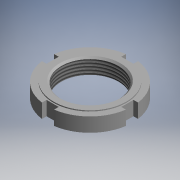
# Autodesk Inventor part: 3753 M30x1.5
Saved by Autodesk Inventor 2017.3 (Build 213256000, 256)
## iProperties
Part Number: 3753 M30x1.5
Material: Generic
Catalog Web Link: www.cadenas.de
Description: NUT-SLOTTED-Slotted nut
Vendor: FESTO
Document SubType Name: Modeling
Designer: partserver
Manufacturer: FESTO
Mass: 5.20156 g
Surface Area: 31.9496 cm^2
Volume: 5.20156 cm^3
Density: 1 g/cm^3
Appearance: PSOLRGB-192-192-192
Category: PARTsolutions
Company: FESTO
Title: 3753 M30x1.5
Author: Cadenas PARTsolutions
Comments: Slotted nut
PSOL_IDENT_0: {$CADENAS_DATA\23d-libs\festo\zyl_zubeh\nutmutter\slotted_nut.prj},169 {VTYP=3D},{NB=3753 M30x1.5},{
PSOL_IDENT_1: LINA=3753 M30x1.5},{NN=NUT-SLOTTED},{DATE=02.10.2018 06:26:15},{GEOMDATE=02.10.2018 06:26:08},{VERSI
PSOL_IDENT_2: ON=},{LINEID=10},{WBVAR=},{WBNUMERIC=}  {NB=3753 M30x1.5},{LINA=3753 M30x1.5},{KT=DUMMY},{TNR=3753},
PSOL_IDENT_3: {TYP=M30x1.5},{D=42.000},{D1=36.000},{DN=30.000},{H=8.000},{H1=2.500},{B=6.000},{P=1.500}
NB: 3753 M30x1.5
NN: NUT-SLOTTED
NT: Slotted nut
NBSYN: $TNR. $TYP.
LINA: 3753 M30x1.5
CATALOG: Festo
TNR: 3753
TYP: M30x1.5
D: 42
D1: 36
DN: 30
H: 8
H1: 2.5
B: 6
P: 1.5
SUPPLIER: FESTO
ARTICLENO: 3753 M30x1.5
BOMINFO: 3753 M30x1.5
CREATOR: CADENAS GmbH
Autodesk Inventor part; units mm, degrees
ref_plane "YZ Plane" through (0, 0, 0) normal (1, 0, 0) x (0, 1, 0)
ref_plane "XZ Plane" through (0, 0, 0) normal (0, 1, 0) x (-1, 0, 0)
ref_plane "XY Plane" through (0, 0, 0) normal (0, 0, 1) x (1, 0, 0)
sketch "Sketch_1" plane through (0, 0, 0) normal (1, 0, 0) x (0, 1, 0)
  line L0 (0, -4) -> (0, 4)
  line L1 (0, 4) -> (18, 4)
  line L2 (18, 4) -> (18, 3.5)
  line L3 (18, 3.5) -> (21, 3.5)
  line L4 (21, 3.5) -> (21, -4)
  line L5 (21, -4) -> (0, -4)
  line L6 (0, -4) -> (0, 4)
  constraints: 14 end point
revolve "Revolution1" add sketch "Sketch_1" angle 360 about axis through (0, 0, -4) along (0, 0, -1)
sketch "Sketch_2" plane through (0, 0, 0) normal (1, 0, 0) x (0, 1, 0)
  line L0 (0, -4) -> (0, 4)
  line L1 (0, 4) -> (15, 4)
  line L2 (15, 4) -> (14.188, 3.5312)
  line L3 (14.188, 3.5312) -> (14.188, -3.188)
  line L4 (14.188, -3.188) -> (15, -4)
  line L5 (15, -4) -> (0, -4)
  line L6 (0, -4) -> (0, 4)
  constraints: 14 end point
revolve "Revolution2" cut sketch "Sketch_2" angle 360 about axis through (0, 0, -4) along (0, 0, -1)
thread "Thread1" size "M30x1.5" class "6H" standard "ISO Metric profile" full length
sketch "Sketch_6" plane through (0, 0, 0) normal (1, 0, 0) x (0, 1, 0)
  line L0 (0, -6) -> (0, -4)
  line L1 (0, -4) -> (18, -4)
  line L2 (18, -4) -> (18, -3.5)
  line L3 (18, -3.5) -> (21, -3.5)
  line L4 (21, -3.5) -> (21, -6)
  line L5 (21, -6) -> (0, -6)
  line L6 (0, -6) -> (0, -4)
  constraints: 14 end point
revolve "Revolution3" cut sketch "Sketch_6" angle 360 about axis through (0, 0, -6) along (0, 0, -1)
sketch "Sketch_3" plane through (0, 0, 0) normal (0, 0, 1) x (1, 0, 0)
  circle A0 centre (0, 0) radius 25.2
  line L0 (-20.7846, 3) -> (-18.5, 3)
  line L1 (-18.5, 3) -> (-18.5, -3)
  line L2 (-18.5, -3) -> (-20.7846, -3)
  arc A1 (-20.7846, -3) -> (-3, -20.7846) centre (0, 0) ccw
  line L3 (-3, -20.7846) -> (-3, -18.5)
  line L4 (-3, -18.5) -> (3, -18.5)
  line L5 (3, -18.5) -> (3, -20.7846)
  arc A2 (3, -20.7846) -> (20.7846, -3) centre (0, 0) ccw
  line L6 (20.7846, -3) -> (18.5, -3)
  line L7 (18.5, -3) -> (18.5, 3)
  line L8 (18.5, 3) -> (20.7846, 3)
  arc A3 (20.7846, 3) -> (3, 20.7846) centre (0, 0) ccw
  line L9 (3, 20.7846) -> (3, 18.5)
  line L10 (3, 18.5) -> (-3, 18.5)
  line L11 (-3, 18.5) -> (-3, 20.7846)
  arc A4 (-3, 20.7846) -> (-20.7846, 3) centre (0, 0) ccw
  constraints: 24 end point, 8 point on circle, 5 centre point
extrude "Extrusion1" cut sketch "Sketch_3" along normal mid plane 8
ref_plane "FDT_CYLINDER_XY" through (0, 0, -4) normal (0, 0, 1) x (1, 0, 0)
ref_plane "FDT_CYLINDER_YZ" through (0, 0, -4) normal (1, 0, 0) x (0, 1, 0)
ref_plane "FDT_CYLINDER_ZX" through (0, 0, -4) normal (0, 1, 0) x (0, 0, 1)
ref_plane "NUT_XY" through (0, 0, 4) normal (0, 0, -1) x (1, 0, 0)
ref_plane "NUT_YZ" through (0, 0, 4) normal (1, 0, 0) x (0, -1, 0)
ref_plane "NUT_ZX" through (0, 0, 4) normal (0, -1, 0) x (0, 0, -1)
body "Solid1"
